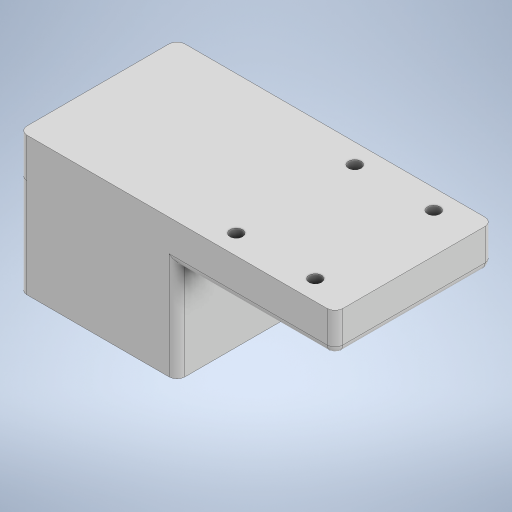
# Autodesk Inventor part: afterdesign
Saved by Autodesk Inventor 2024 (Build 280153000, 153)
## iProperties
Created: 2025-05-07
Part Number: afterdesign
Material: Generic
Document SubType Name: Modeling
Designer: Bjarni Heselmans
Density: 1 g/cm^3
Appearance: Default
Author: Bjarni Heselmans
Autodesk Inventor part; units mm, degrees
ref_plane "YZ Plane" through (0, 0, 0) normal (1, 0, 0) x (0, 1, 0)
ref_plane "XZ Plane" through (0, 0, 0) normal (0, 1, 0) x (-1, 0, 0)
ref_plane "XY Plane" through (0, 0, 0) normal (0, 0, 1) x (1, 0, 0)
sketch "Sketch1" plane through (0, 0, 0) normal (0, 0, 1) x (1, 0, 0)
  arc A0 (-1.9978, -1.5) -> (-1.9978, 1.5) centre (0.0022, 0) ccw
  line L0 (2.5022, 0) -> (-1.9978, 0)
  line L1 (-1.9978, 0) -> (-1.9978, 1.5)
  line L2 (-1.9978, 0) -> (-1.9978, -1.5)
  line L3 (0.0022, 0) -> (20.0022, 0)
  line L4 (0.0022, 0) -> (0.0022, -20)
  line L5 (18.0022, -20) -> (-17.9978, -20)
  line L6 (-19.9978, -18) -> (-19.9978, 18)
  line L7 (-17.9978, 20) -> (18.0022, 20)
  line L8 (20.0022, 18) -> (20.0022, -18)
  line L9 (14.4, 14.4) -> (14.4, 20)
  line L10 (20.0022, 14.4) -> (16.0022, 14.4)
  circle A1 centre (14.4, 14.4) radius 1.6022
  circle A2 centre (14.4, -14.4) radius 1.6022
  circle A3 centre (-14.3955, 14.4) radius 1.6022
  circle A4 centre (-14.3955, -14.4) radius 1.6022
  arc A5 (-17.9978, 20) -> (-19.9978, 18) centre (-17.9978, 18) ccw
  arc A6 (20.0022, 18) -> (18.0022, 20) centre (18.0022, 18) ccw
  arc A7 (18.0022, -20) -> (20.0022, -18) centre (18.0022, -18) ccw
  arc A8 (-19.9978, -18) -> (-17.9978, -20) centre (-17.9978, -18) ccw
  point P0 (0, 0)
  point P1 (0.2522, 0)
  point P2 (-1.9978, 0.75)
  point P3 (-19.9978, 20)
  point P4 (-19.9978, -20)
  point P5 (20.0022, 20)
  dimension "d0" = 5
  dimension "d1" = 4.5
  dimension "d21" = 20
  dimension "d22" = 20
  dimension "d23" = 40
  dimension "d24" = 40
  dimension "d25" = 20
  dimension "d26" = 5.6
  dimension "d27" = 4
  dimension "d28" = 2
  constraints: 22 end point, 11 point on circle, 10 point on line, 8 centre point, 8 tangent, 3 equal radius, 3 horizontal, 3 symmetric about line, 2 coincident, 2 midpoint, 2 parallel, 2 perpendicular, 2 vertical, 1 horizontal alignment, 5 other
  measures "d0" diameter of A0
  measures "d1" distance of L0.start L0.end
  measures "d21" distance of L3.start L3.end
  measures "d22" distance of L3.start L4.end
  measures "d23" distance of point (-19.998, 20) point (20.002, 20)
  measures "d24" distance of point (-19.998, -20) point (-19.998, 20)
  measures "d25" distance from line of point (0.002, 0) L7
  measures "d26" distance from line of L9.start L7
  measures "d27" distance of L10.start L10.end
  measures "d28" radius of A5
extrude "Extrusion1" add sketch "Sketch1" along normal blind 25 contours L3 L8 A7 L5 L4 A0 | A0 L1 L2 L4 L5 A8 L6 A5 L7 L9 A1 L10 L8 L3 | L10 A1 L9 L7 A6 L8
sketch "Sketch2" plane through (-19.9978, -18, 0) normal (-1, 0, 0) x (0, 0, 1)
  line L0 (0, 38) -> (25, 38) projected
  line L1 (0, 38) -> (12.5, 38)
  line L2 (12.5, 38) -> (12.5, 19.625)
  line L3 (12.5, 18) -> (0, 18)
  line L4 (0, 18) -> (0, 38)
  circle A0 centre (12.5, 18) radius 1.625
  dimension "d33" = 3.25
  dimension "d31" = 12.5
  dimension "d32" = 20
  constraints: 8 end point, 2 parallel, 1 coincident, 1 horizontal, 1 perpendicular, 1 vertical alignment, 2 other
  measures "d31" distance of L3.start L3.end
  measures "d32" distance of L1.end L3.start
extrude "Extrusion2" cut sketch "Sketch2" against normal blind 20 contours A0
sketch "Sketch3" plane through (0, 0, 25) normal (0, 0, 1) x (1, 0, 0)
  line L0 (58, -20) -> (-18, -20)
  line L1 (-20, -18) -> (-20, 18)
  line L2 (-18, 20) -> (58, 20)
  line L3 (60, 18) -> (60, -18)
  arc A0 (58, -20) -> (60, -18) centre (58, -18) ccw
  arc A1 (60, 18) -> (58, 20) centre (58, 18) ccw
  arc A2 (-18, 20) -> (-20, 18) centre (-18, 18) ccw
  arc A3 (-20, -18) -> (-18, -20) centre (-18, -18) ccw
  point P0 (0, 0)
  dimension "d36" = 60
  dimension "d37" = 20
  dimension "d38" = 20
  dimension "d39" = 20
  dimension "d40" = 2
  constraints: 8 end point, 8 point on circle, 8 tangent, 4 centre point, 3 equal radius, 2 parallel, 1 horizontal, 1 perpendicular
  measures "d36" distance from line of point (0, 0) L3
  measures "d37" distance from line of point (0, 0) L0
  measures "d38" distance from line of point (0, 0) L1
  measures "d39" distance from line of point (0, 0) L2
  measures "d40" radius of A0
extrude "Extrusion3" add sketch "Sketch3" along normal blind 10
sketch "Sketch7" plane through (0, 0, 35) normal (0, 0, 1) x (1, 0, 0)
  line L0 (55.0022, 20) -> (50.0022, 20)
  line L1 (50.0022, 20) -> (50.0022, 15)
  line L2 (50.0022, 15) -> (55.0022, 15)
  line L3 (55.0022, 15) -> (55.0022, 20)
  circle A0 centre (50.0022, 15) radius 1.6
  line L4 (18.0022, 20) -> (-17.9978, 20) projected
  line L5 (0.0022, 20) -> (60.0022, 20)
  line L6 (60.0022, 20) -> (60.0022, -20)
  line L7 (60.0022, -20) -> (0.0022, -20)
  line L8 (0.0022, -20) -> (0.0022, 20)
  circle A1 centre (50.0022, -15) radius 1.6
  line L9 (60.0022, -20) -> (20.0022, -20)
  line L10 (20.0022, -20) -> (20.0022, 20)
  line L11 (20.0022, 20) -> (60.0022, 20)
  line L12 (60.0022, 20) -> (60.0022, -20)
  line L13 (58, 20) -> (-18, 20) projected
  line L14 (40.0022, 20) -> (40.0022, -20)
  circle A2 centre (30.0022, 15) radius 1.6
  circle A3 centre (30.0022, -15) radius 1.6
  point P0 (0, 0)
  dimension "d73" = 5
  dimension "d74" = 5
  dimension "d75" = 3.2
  dimension "d78" = 60
  dimension "d81" = 60
  dimension "d85" = 40
  dimension "d86" = 30
  dimension "d87" = 20
  constraints: 26 end point, 6 parallel, 4 centre point, 3 horizontal, 3 perpendicular, 2 midpoint, 2 point on line, 2 symmetric about line, 1 coincident, 2 other
  measures "d73" distance of L2.end L1.end
  measures "d74" distance of L1.end L0.end
  measures "d75" diameter of A0
  measures "d78" distance between parallel lines of L6 L8
  measures "d81" distance of L5.start L5.end
  measures "d85" distance of L10.end L11.end
  measures "d86" distance of A1.centre L1.end
  measures "d87" distance of A2.centre L1.end
extrude "Extrusion6" cut sketch "Sketch7" against normal blind 20 contours A0 L2 L1 | L1 L2 A0 | A1 | A2 | A3
fillet "Fillet3" radius 2 5 edges at (59.4142, -19.4142, 25) (60, 0, 25) (59.4142, 19.4142, 25) (38.0011, 20, 25) (38.0011, -20, 25)
body "Solid1"
